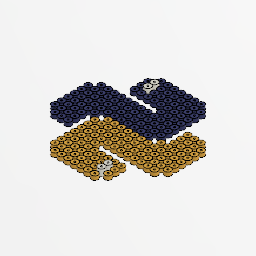
fusion (Autodesk Fusion 360 design; units mm, degrees)
Autodesk Fusion 360 part; units mm, degrees
sketch "Sketch1" plane through (0, 0, 0) normal (0, 0, 1) x (1, 0, 0)
  circle A0 centre (0, 0) radius 2.5
  circle A1 centre (0, 0) radius 0.65
  circle A2 centre (-5, 0) radius 0.65
  circle A3 centre (-5, 0) radius 2.5
  circle A4 centre (-10, 0) radius 0.65
  circle A5 centre (-10, 0) radius 2.5
  circle A6 centre (-10, 5) radius 2.5
  circle A7 centre (-10, 5) radius 0.65
  circle A8 centre (-5, 5) radius 0.65
  circle A9 centre (0, 5) radius 0.65
  circle A10 centre (-5, 5) radius 2.5
  circle A11 centre (0, 5) radius 2.5
  circle A12 centre (-10, 10) radius 2.5
  circle A13 centre (-10, 10) radius 0.65
  circle A14 centre (-5, 10) radius 0.65
  circle A15 centre (0, 10) radius 0.65
  circle A16 centre (-5, 10) radius 2.5
  circle A17 centre (0, 10) radius 2.5
  circle A18 centre (-10, 15) radius 2.5
  circle A19 centre (-10, 15) radius 0.65
  circle A20 centre (-5, 15) radius 0.65
  circle A21 centre (0, 15) radius 0.65
  circle A22 centre (-5, 15) radius 2.5
  circle A23 centre (0, 15) radius 2.5
  circle A24 centre (-10, 20) radius 2.5
  circle A25 centre (-10, 20) radius 0.65
  circle A26 centre (-5, 20) radius 0.65
  circle A27 centre (0, 20) radius 0.65
  circle A28 centre (-5, 20) radius 2.5
  circle A29 centre (0, 20) radius 2.5
  circle A30 centre (-10, 25) radius 2.5
  circle A31 centre (-10, 25) radius 0.65
  circle A32 centre (-5, 25) radius 0.65
  circle A33 centre (0, 25) radius 0.65
  circle A34 centre (-5, 25) radius 2.5
  circle A35 centre (0, 25) radius 2.5
  circle A36 centre (-10, 30) radius 2.5
  circle A37 centre (-10, 30) radius 0.65
  circle A38 centre (-5, 30) radius 0.65
  circle A39 centre (0, 30) radius 0.65
  circle A40 centre (-5, 30) radius 2.5
  circle A41 centre (0, 30) radius 2.5
  circle A42 centre (-10, 35) radius 2.5
  circle A43 centre (-10, 35) radius 0.65
  circle A44 centre (-5, 35) radius 0.65
  circle A45 centre (0, 35) radius 0.65
  circle A46 centre (-5, 35) radius 2.5
  circle A47 centre (0, 35) radius 2.5
  circle A48 centre (-15, 30) radius 0.65
  circle A49 centre (-15, 25) radius 0.65
  circle A50 centre (-15, 5) radius 0.65
  circle A51 centre (-15, 10) radius 0.65
  circle A52 centre (-15, 20) radius 0.65
  circle A53 centre (-15, 15) radius 0.65
  circle A54 centre (-15, 30) radius 2.5
  circle A55 centre (-15, 25) radius 2.5
  circle A56 centre (-15, 20) radius 2.5
  circle A57 centre (-15, 15) radius 2.5
  circle A58 centre (-15, 10) radius 2.5
  circle A59 centre (-15, 5) radius 2.5
  circle A60 centre (5, 20) radius 2.5
  circle A61 centre (5, 15) radius 0.65
  circle A62 centre (5, 30) radius 2.5
  circle A63 centre (5, 35) radius 2.5
  circle A64 centre (5, 25) radius 0.65
  circle A65 centre (5, 15) radius 2.5
  circle A66 centre (5, 25) radius 2.5
  circle A67 centre (5, 30) radius 0.65
  circle A68 centre (5, 20) radius 0.65
  circle A69 centre (5, 35) radius 0.65
  circle A70 centre (10, 30) radius 2.5
  circle A71 centre (10, 35) radius 2.5
  circle A72 centre (10, 20) radius 2.5
  circle A73 centre (10, 30) radius 0.65
  circle A74 centre (10, 35) radius 0.65
  circle A75 centre (10, 25) radius 0.65
  circle A76 centre (10, 20) radius 0.65
  circle A77 centre (10, 25) radius 2.5
  circle A78 centre (15, 30) radius 2.5
  circle A79 centre (15, 35) radius 2.5
  circle A80 centre (15, 20) radius 2.5
  circle A81 centre (15, 30) radius 0.65
  circle A82 centre (15, 35) radius 0.65
  circle A83 centre (15, 25) radius 0.65
  circle A84 centre (15, 20) radius 0.65
  circle A85 centre (15, 25) radius 2.5
  circle A86 centre (20, 30) radius 2.5
  circle A87 centre (20, 35) radius 2.5
  circle A88 centre (20, 20) radius 2.5
  circle A89 centre (20, 30) radius 0.65
  circle A90 centre (20, 35) radius 0.65
  circle A91 centre (20, 25) radius 0.65
  circle A92 centre (20, 20) radius 0.65
  circle A93 centre (20, 25) radius 2.5
  circle A94 centre (25, 30) radius 2.5
  circle A95 centre (25, 35) radius 2.5
  circle A96 centre (25, 20) radius 2.5
  circle A97 centre (25, 30) radius 0.65
  circle A98 centre (25, 35) radius 0.65
  circle A99 centre (25, 25) radius 0.65
  circle A100 centre (25, 20) radius 0.65
  circle A101 centre (25, 25) radius 2.5
  circle A102 centre (30, 30) radius 2.5
  circle A103 centre (30, 35) radius 2.5
  circle A104 centre (30, 20) radius 2.5
  circle A105 centre (30, 30) radius 0.65
  circle A106 centre (30, 35) radius 0.65
  circle A107 centre (30, 25) radius 0.65
  circle A108 centre (30, 20) radius 0.65
  circle A109 centre (30, 25) radius 2.5
  circle A110 centre (35, 30) radius 2.5
  circle A111 centre (35, 35) radius 2.5
  circle A112 centre (35, 20) radius 2.5
  circle A113 centre (35, 30) radius 0.65
  circle A114 centre (35, 35) radius 0.65
  circle A115 centre (35, 25) radius 0.65
  circle A116 centre (35, 20) radius 0.65
  circle A117 centre (35, 25) radius 2.5
  circle A118 centre (40, 30) radius 2.5
  circle A119 centre (40, 35) radius 2.5
  circle A120 centre (40, 20) radius 2.5
  circle A121 centre (40, 30) radius 0.65
  circle A122 centre (40, 35) radius 0.65
  circle A123 centre (40, 25) radius 0.65
  circle A124 centre (40, 20) radius 0.65
  circle A125 centre (40, 25) radius 2.5
  circle A126 centre (45, 30) radius 2.5
  circle A127 centre (45, 35) radius 2.5
  circle A128 centre (45, 30) radius 0.65
  circle A129 centre (45, 35) radius 0.65
  circle A130 centre (45, 25) radius 0.65
  circle A131 centre (45, 25) radius 2.5
  circle A132 centre (40, 40) radius 0.65
  circle A133 centre (40, 40) radius 2.5
  circle A134 centre (35, 40) radius 2.5
  circle A135 centre (45, 40) radius 0.65
  circle A136 centre (45, 40) radius 2.5
  circle A137 centre (30, 40) radius 0.65
  circle A138 centre (35, 40) radius 0.65
  circle A139 centre (30, 40) radius 2.5
  circle A140 centre (40, 45) radius 0.65
  circle A141 centre (40, 45) radius 2.5
  circle A142 centre (35, 45) radius 2.5
  circle A143 centre (45, 45) radius 0.65
  circle A144 centre (45, 45) radius 2.5
  circle A145 centre (30, 45) radius 0.65
  circle A146 centre (35, 45) radius 0.65
  circle A147 centre (30, 45) radius 2.5
  circle A148 centre (40, 50) radius 0.65
  circle A149 centre (40, 50) radius 2.5
  circle A150 centre (35, 50) radius 2.5
  circle A151 centre (45, 50) radius 0.65
  circle A152 centre (45, 50) radius 2.5
  circle A153 centre (30, 50) radius 0.65
  circle A154 centre (35, 50) radius 0.65
  circle A155 centre (30, 50) radius 2.5
  circle A156 centre (40, 55) radius 0.65
  circle A157 centre (40, 55) radius 2.5
  circle A158 centre (35, 55) radius 2.5
  circle A159 centre (45, 55) radius 0.65
  circle A160 centre (45, 55) radius 2.5
  circle A161 centre (30, 55) radius 0.65
  circle A162 centre (35, 55) radius 0.65
  circle A163 centre (30, 55) radius 2.5
  circle A164 centre (40, 60) radius 0.65
  circle A165 centre (40, 60) radius 2.5
  circle A166 centre (35, 60) radius 2.5
  circle A167 centre (30, 60) radius 0.65
  circle A168 centre (35, 60) radius 0.65
  circle A169 centre (30, 60) radius 2.5
  circle A170 centre (25, 60) radius 0.65
  circle A171 centre (25, 45) radius 0.65
  circle A172 centre (25, 55) radius 0.65
  circle A173 centre (25, 55) radius 2.5
  circle A174 centre (25, 50) radius 2.5
  circle A175 centre (25, 60) radius 2.5
  circle A176 centre (25, 45) radius 2.5
  circle A177 centre (25, 50) radius 0.65
  circle A178 centre (20, 60) radius 0.65
  circle A179 centre (20, 45) radius 0.65
  circle A180 centre (20, 55) radius 0.65
  circle A181 centre (20, 55) radius 2.5
  circle A182 centre (20, 50) radius 2.5
  circle A183 centre (20, 60) radius 2.5
  circle A184 centre (20, 45) radius 2.5
  circle A185 centre (20, 50) radius 0.65
  circle A186 centre (15, 60) radius 0.65
  circle A187 centre (15, 45) radius 0.65
  circle A188 centre (15, 55) radius 0.65
  circle A189 centre (15, 55) radius 2.5
  circle A190 centre (15, 50) radius 2.5
  circle A191 centre (15, 60) radius 2.5
  circle A192 centre (15, 45) radius 2.5
  circle A193 centre (15, 50) radius 0.65
  circle A194 centre (10, 60) radius 0.65
  circle A195 centre (10, 45) radius 0.65
  circle A196 centre (10, 55) radius 0.65
  circle A197 centre (10, 55) radius 2.5
  circle A198 centre (10, 50) radius 2.5
  circle A199 centre (10, 60) radius 2.5
  circle A200 centre (10, 45) radius 2.5
  circle A201 centre (10, 50) radius 0.65
  circle A202 centre (5, 50) radius 2.5
  circle A203 centre (5, 45) radius 2.5
  circle A204 centre (5, 50) radius 0.65
  circle A205 centre (5, 55) radius 2.5
  circle A206 centre (5, 55) radius 0.65
  circle A207 centre (5, 45) radius 0.65
  circle A208 centre (15, -5) radius 0.65
  circle A209 centre (35, -20) radius 2.5
  circle A210 centre (45, -15) radius 2.5
  circle A211 centre (35, 10) radius 2.5
  circle A212 centre (50, 0) radius 0.65
  circle A213 centre (45, -20) radius 0.65
  circle A214 centre (60, 30) radius 0.65
  circle A215 centre (35, 5) radius 0.65
  circle A216 centre (45, 5) radius 0.65
  circle A217 centre (45, 10) radius 0.65
  circle A218 centre (50, 15) radius 2.5
  circle A219 centre (30, 0) radius 0.65
  circle A220 centre (35, 0) radius 2.5
  circle A221 centre (25, -5) radius 0.65
  circle A222 centre (20, -20) radius 0.65
  circle A223 centre (60, 35) radius 0.65
  circle A224 centre (10, -15) radius 2.5
  circle A225 centre (20, -20) radius 2.5
  circle A226 centre (40, -10) radius 2.5
  circle A227 centre (40, 15) radius 0.65
  circle A228 centre (65, 30) radius 2.5
  circle A229 centre (65, 35) radius 0.65
  circle A230 centre (20, -15) radius 0.65
  circle A231 centre (30, 10) radius 0.65
  circle A232 centre (15, -10) radius 0.65
  circle A233 centre (60, 30) radius 2.5
  circle A234 centre (15, 15) radius 2.5
  circle A235 centre (20, 0) radius 2.5
  circle A236 centre (15, 5) radius 2.5
  circle A237 centre (55, 25) radius 2.5
  circle A238 centre (45, 15) radius 0.65
  circle A239 centre (40, 5) radius 2.5
  circle A240 centre (50, -15) radius 2.5
  circle A241 centre (55, 5) radius 0.65
  circle A242 centre (35, -20) radius 0.65
  circle A243 centre (45, -15) radius 0.65
  circle A244 centre (25, -15) radius 0.65
  circle A245 centre (10, 0) radius 2.5
  circle A246 centre (30, -15) radius 0.65
  circle A247 centre (40, -15) radius 2.5
  circle A248 centre (20, 0) radius 0.65
  circle A249 centre (35, -10) radius 0.65
  circle A250 centre (40, -15) radius 0.65
  circle A251 centre (15, -20) radius 2.5
  circle A252 centre (40, -10) radius 0.65
  circle A253 centre (70, 30) radius 2.5
  circle A254 centre (20, 5) radius 0.65
  circle A255 centre (30, 5) radius 2.5
  circle A256 centre (35, 0) radius 0.65
  circle A257 centre (15, 5) radius 0.65
  circle A258 centre (25, 5) radius 2.5
  circle A259 centre (15, -15) radius 0.65
  circle A260 centre (10, -15) radius 0.65
  circle A261 centre (15, -20) radius 0.65
  circle A262 centre (35, 5) radius 2.5
  circle A263 centre (40, -25) radius 0.65
  circle A264 centre (45, 0) radius 0.65
  circle A265 centre (65, 10) radius 0.65
  circle A266 centre (15, -15) radius 2.5
  circle A267 centre (40, -20) radius 2.5
  circle A268 centre (30, 0) radius 2.5
  circle A269 centre (25, 0) radius 2.5
  circle A270 centre (10, -5) radius 2.5
  circle A271 centre (15, 0) radius 2.5
  circle A272 centre (70, 5) radius 2.5
  circle A273 centre (15, 15) radius 0.65
  circle A274 centre (50, -10) radius 0.65
  circle A275 centre (60, 10) radius 0.65
  circle A276 centre (25, -20) radius 0.65
  circle A277 centre (10, 5) radius 2.5
  circle A278 centre (40, 10) radius 0.65
  circle A279 centre (20, 10) radius 2.5
  circle A280 centre (20, -5) radius 0.65
  circle A281 centre (35, 10) radius 0.65
  circle A282 centre (20, -25) radius 2.5
  circle A283 centre (30, 15) radius 2.5
  circle A284 centre (35, -15) radius 0.65
  circle A285 centre (50, 15) radius 0.65
  circle A286 centre (30, 5) radius 0.65
  circle A287 centre (40, 15) radius 2.5
  circle A288 centre (15, -10) radius 2.5
  circle A289 centre (30, -15) radius 2.5
  circle A290 centre (60, 35) radius 2.5
  circle A291 centre (50, 5) radius 2.5
  circle A292 centre (50, -20) radius 2.5
  circle A293 centre (20, -5) radius 2.5
  circle A294 centre (10, -5) radius 0.65
  circle A295 centre (65, 35) radius 2.5
  circle A296 centre (10, -20) radius 0.65
  circle A297 centre (70, 25) radius 0.65
  circle A298 centre (70, 20) radius 2.5
  circle A299 centre (55, 10) radius 2.5
  circle A300 centre (15, 0) radius 0.65
  circle A301 centre (55, 15) radius 0.65
  circle A302 centre (25, -5) radius 2.5
  circle A303 centre (15, 10) radius 2.5
  circle A304 centre (20, -15) radius 2.5
  circle A305 centre (10, 10) radius 2.5
  circle A306 centre (30, 10) radius 2.5
  circle A307 centre (35, -15) radius 2.5
  circle A308 centre (55, 0) radius 2.5
  circle A309 centre (60, 5) radius 2.5
  circle A310 centre (65, 30) radius 0.65
  circle A311 centre (50, 10) radius 0.65
  circle A312 centre (70, 10) radius 0.65
  circle A313 centre (65, 5) radius 0.65
  circle A314 centre (25, -20) radius 2.5
  circle A315 centre (20, 10) radius 0.65
  circle A316 centre (45, 15) radius 2.5
  circle A317 centre (25, -10) radius 0.65
  circle A318 centre (25, -15) radius 2.5
  circle A319 centre (65, 10) radius 2.5
  circle A320 centre (10, 0) radius 0.65
  circle A321 centre (35, -25) radius 2.5
  circle A322 centre (60, 10) radius 2.5
  circle A323 centre (35, 15) radius 0.65
  circle A324 centre (70, 15) radius 0.65
  circle A325 centre (55, 15) radius 2.5
  circle A326 centre (25, 15) radius 0.65
  circle A327 centre (50, -10) radius 2.5
  circle A328 centre (60, 0) radius 0.65
  circle A329 centre (15, 10) radius 0.65
  circle A330 centre (30, -20) radius 0.65
  circle A331 centre (10, 10) radius 0.65
  circle A332 centre (60, 5) radius 0.65
  circle A333 centre (55, 0) radius 0.65
  circle A334 centre (25, 15) radius 2.5
  circle A335 centre (70, 15) radius 2.5
  circle A336 centre (60, 0) radius 2.5
  circle A337 centre (20, -10) radius 2.5
  circle A338 centre (65, 0) radius 0.65
  circle A339 centre (55, 5) radius 2.5
  circle A340 centre (40, 10) radius 2.5
  circle A341 centre (30, -20) radius 2.5
  circle A342 centre (30, -10) radius 2.5
  circle A343 centre (55, 30) radius 0.65
  circle A344 centre (15, -5) radius 2.5
  circle A345 centre (25, 5) radius 0.65
  circle A346 centre (65, 25) radius 2.5
  circle A347 centre (15, -25) radius 0.65
  circle A348 centre (25, 10) radius 0.65
  circle A349 centre (65, 5) radius 2.5
  circle A350 centre (60, 20) radius 0.65
  circle A351 centre (20, -25) radius 0.65
  circle A352 centre (30, -25) radius 2.5
  circle A353 centre (65, 15) radius 0.65
  circle A354 centre (10, 5) radius 0.65
  circle A355 centre (45, 5) radius 2.5
  circle A356 centre (40, 0) radius 0.65
  circle A357 centre (50, 20) radius 2.5
  circle A358 centre (30, -25) radius 0.65
  circle A359 centre (70, 20) radius 0.65
  circle A360 centre (45, -25) radius 0.65
  circle A361 centre (20, 15) radius 2.5
  circle A362 centre (70, 25) radius 2.5
  circle A363 centre (70, 5) radius 0.65
  circle A364 centre (60, 15) radius 2.5
  circle A365 centre (50, 0) radius 2.5
  circle A366 centre (45, 10) radius 2.5
  circle A367 centre (50, -20) radius 0.65
  circle A368 centre (60, 25) radius 0.65
  circle A369 centre (55, 35) radius 2.5
  circle A370 centre (20, 15) radius 0.65
  circle A371 centre (45, -10) radius 2.5
  circle A372 centre (40, 0) radius 2.5
  circle A373 centre (55, 20) radius 0.65
  circle A374 centre (45, -10) radius 0.65
  circle A375 centre (40, 5) radius 0.65
  circle A376 centre (45, 0) radius 2.5
  circle A377 centre (65, 15) radius 2.5
  circle A378 centre (60, 15) radius 0.65
  circle A379 centre (30, -10) radius 0.65
  circle A380 centre (55, 35) radius 0.65
  circle A381 centre (25, -10) radius 2.5
  circle A382 centre (45, -25) radius 2.5
  circle A383 centre (65, 20) radius 2.5
  circle A384 centre (55, 25) radius 0.65
  circle A385 centre (15, -25) radius 2.5
  circle A386 centre (65, 20) radius 0.65
  circle A387 centre (55, 10) radius 0.65
  circle A388 centre (25, -25) radius 0.65
  circle A389 centre (70, 30) radius 0.65
  circle A390 centre (55, 20) radius 2.5
  circle A391 centre (40, -20) radius 0.65
  circle A392 centre (65, 25) radius 0.65
  circle A393 centre (50, 5) radius 0.65
  circle A394 centre (35, -10) radius 2.5
  circle A395 centre (35, 15) radius 2.5
  circle A396 centre (55, 30) radius 2.5
  circle A397 centre (45, -20) radius 2.5
  circle A398 centre (40, -25) radius 2.5
  circle A399 centre (60, 20) radius 2.5
  circle A400 centre (30, 15) radius 0.65
  circle A401 centre (35, -25) radius 0.65
  circle A402 centre (50, 20) radius 0.65
  circle A403 centre (70, 10) radius 2.5
  circle A404 centre (25, 0) radius 0.65
  circle A405 centre (25, -25) radius 2.5
  circle A406 centre (65, 0) radius 2.5
  circle A407 centre (50, -15) radius 0.65
  circle A408 centre (50, 10) radius 2.5
  circle A409 centre (25, 10) radius 2.5
  circle A410 centre (20, 5) radius 2.5
  circle A411 centre (60, 25) radius 2.5
  circle A412 centre (20, -10) radius 0.65
  circle A413 centre (10, -10) radius 2.5
  circle A414 centre (10, -20) radius 2.5
  circle A415 centre (10, -10) radius 0.65
  point P0 (0, 5)
  point P1 (0, 10)
  point P2 (0, 15)
  point P3 (0, 20)
  point P4 (0, 25)
  point P5 (0, 30)
  point P6 (0, 35)
  point P7 (5, 35)
  point P8 (5, 30)
  point P9 (5, 25)
  point P10 (5, 15)
  point P11 (5, 20)
  point P12 (10, 30)
  point P13 (10, 25)
  point P14 (10, 20)
  point P15 (10, 35)
  point P16 (15, 30)
  point P17 (15, 25)
  point P18 (15, 20)
  point P19 (15, 35)
  point P20 (20, 30)
  point P21 (20, 25)
  point P22 (20, 20)
  point P23 (20, 35)
  point P24 (25, 30)
  point P25 (25, 25)
  point P26 (25, 20)
  point P27 (25, 35)
  point P28 (30, 30)
  point P29 (30, 25)
  point P30 (30, 20)
  point P31 (30, 35)
  point P32 (35, 30)
  point P33 (35, 25)
  point P34 (35, 20)
  point P35 (35, 35)
  point P36 (40, 30)
  point P37 (40, 25)
  point P38 (40, 20)
  point P39 (40, 35)
  point P40 (45, 30)
  point P41 (45, 25)
  point P42 (45, 35)
  point P43 (45, 40)
  point P44 (30, 40)
  point P45 (35, 40)
  point P46 (40, 40)
  point P47 (45, 45)
  point P48 (30, 45)
  point P49 (35, 45)
  point P50 (40, 45)
  point P51 (45, 50)
  point P52 (30, 50)
  point P53 (35, 50)
  point P54 (40, 50)
  point P55 (45, 55)
  point P56 (30, 55)
  point P57 (35, 55)
  point P58 (40, 55)
  point P59 (30, 60)
  point P60 (35, 60)
  point P61 (40, 60)
  point P62 (25, 45)
  point P63 (25, 60)
  point P64 (25, 55)
  point P65 (25, 50)
  point P66 (20, 45)
  point P67 (20, 60)
  point P68 (20, 55)
  point P69 (20, 50)
  point P70 (15, 45)
  point P71 (15, 60)
  point P72 (15, 55)
  point P73 (15, 50)
  point P74 (10, 45)
  point P75 (10, 60)
  point P76 (10, 55)
  point P77 (10, 50)
  point P78 (5, 45)
  point P79 (5, 55)
  point P80 (5, 50)
  point P81 (45, 15)
  point P82 (15, -15)
  point P83 (10, -20)
  point P84 (40, 15)
  point P85 (30, 15)
  point P86 (20, 15)
  point P87 (55, 25)
  point P88 (55, 5)
  point P89 (30, -10)
  point P90 (20, 0)
  point P91 (25, 5)
  point P92 (35, -15)
  point P93 (30, 10)
  point P94 (40, -20)
  point P95 (20, -15)
  point P96 (50, 15)
  point P97 (30, 5)
  point P98 (25, 10)
  point P99 (50, -10)
  point P100 (25, 0)
  point P101 (10, 10)
  point P102 (35, 5)
  point P103 (35, -10)
  point P104 (15, 10)
  point P105 (15, -25)
  point P106 (50, 0)
  point P107 (35, -25)
  point P108 (20, -5)
  point P109 (20, -20)
  point P110 (50, 5)
  point P111 (50, 10)
  point P112 (15, -20)
  point P113 (40, -10)
  point P114 (55, 0)
  point P115 (40, -25)
  point P116 (25, 15)
  point P117 (20, -25)
  point P118 (55, 20)
  point P119 (25, -10)
  point P120 (30, -25)
  point P121 (15, 0)
  point P122 (55, 10)
  point P123 (40, 5)
  point P124 (50, -20)
  point P125 (40, 0)
  point P126 (35, -20)
  point P127 (25, -15)
  point P128 (45, 5)
  point P129 (15, -10)
  point P130 (45, -15)
  point P131 (40, -15)
  point P132 (30, -15)
  point P133 (20, -10)
  point P134 (10, -10)
  point P135 (10, 0)
  point P136 (50, 20)
  point P137 (55, 15)
  point P138 (50, -15)
  point P139 (10, -15)
  point P140 (30, -20)
  point P141 (10, -5)
  point P142 (15, -5)
  point P143 (15, 15)
  point P144 (35, 15)
  point P145 (35, 10)
  point P146 (45, 10)
  point P147 (20, 5)
  point P148 (55, 35)
  point P149 (35, 0)
  point P150 (45, 0)
  point P151 (55, 30)
  point P152 (20, 10)
  point P153 (45, -25)
  point P154 (30, 0)
  point P155 (25, -20)
  point P156 (15, 5)
  point P157 (40, 10)
  point P158 (10, 5)
  point P159 (25, -5)
  point P160 (45, -20)
  point P161 (45, -10)
  point P162 (25, -25)
  dimension "d1" = 5
  dimension "d2" = 1.3
  dimension "d15" = -5
  dimension "d16" = 0
  dimension "d19" = 5
  dimension "d20" = 0
  dimension "d23" = 40
  dimension "d24" = 0
  dimension "d27" = 0
  dimension "d28" = 5
  dimension "d31" = -5
  dimension "d32" = 0
  dimension "d35" = -5
  dimension "d36" = 0
  measures "d1" diameter of A0
  measures "d2" diameter of A1
extrude "Extrude2" add sketch "Sketch1" along normal blind 3 contours A0 | A3 | A11 | A5 | A10 | A6 | A16 | A17 | A59 | A12 | A58 | A18 | A22 | A23 | A57 | A65 | A56 | A24 | A28 | A29 | A60 | A55 | A72 | A54 | A30 | A34 | A35 | A66 | A80 | A77 | A36 | A85 | A42 | A40 | A41 | A62 | A70 | A88 | A93 | A78 | A46 | A86 | A47 | A63 | A71 | A79 | A96 | A101 | A94 | A87 | A95 | A104 | A109 | A102 | A103 | A139 | A112 | A117 | A110 | A111 | A147 | A134 | A176 | A142 | A120 | A125 | A118 | A119 | A133 | A155 | A184 | A174 | A150 | A141 | A192 | A182 | A149 | A131 | A126 | A127 | A136 | A144 | A163 | A173 | A158 | A200 | A190 | A181 | A157 | A152 | A203 | A189 | A160 | A169 | A175 | A166 | A183 | A165 | A202 | A191 | A205 | A199 makes body 1
extrude "Extrude3" add sketch "Sketch1" along normal blind 3 separate body contours A234 | A361 | A303 | A279 | A305 | A334 | A409 | A410 | A236 | A277 | A258 | A245 | A283 | A306 | A255 | A269 | A235 | A271 | A270 | A268 | A344 | A413 | A395 | A211 | A262 | A220 | A302 | A293 | A288 | A224 | A372 | A337 | A266 | A414 | A287 | A340 | A239 | A376 | A381 | A304 | A251 | A365 | A355 | A342 | A318 | A225 | A385 | A316 | A366 | A308 | A291 | A394 | A289 | A314 | A282 | A218 | A336 | A339 | A408 | A226 | A307 | A341 | A405 | A357 | A406 | A309 | A299 | A371 | A247 | A209 | A352 | A325 | A390 | A349 | A322 | A327 | A267 | A321 | A237 | A272 | A319 | A364 | A240 | A398 | A399 | A396 | A411 | A403 | A377 | A292 | A382 | A369 | A233 | A335 | A383 | A346 | A290 | A228 | A298 | A295 | A362 | A253 makes body 2
extrude "Extrude4" add sketch "Sketch1" along normal blind 5 separate body contours A198 | A197 | A210 | A397 makes body 3 at (7.6508, 49.1449, 3.3333) makes body 3 at (12.3492, 55.8551, 3.3333) makes body 4 at (47.3492, -14.1449, 3.3333) makes body 4 at (43.0072, -21.5095, 3.3333)
named bodies: "Blue", "Yellow", "White1", "White2"
